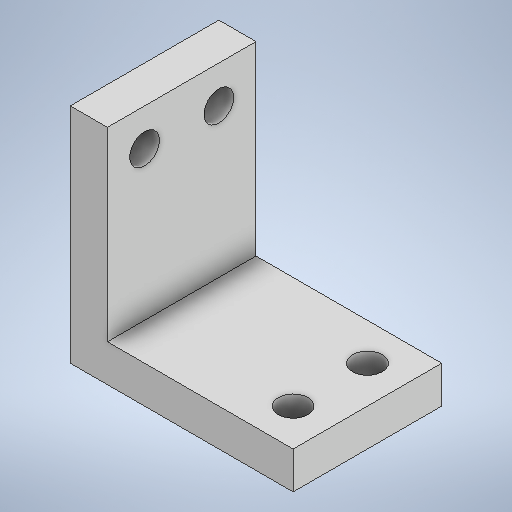
# Autodesk Inventor part: Fastener
Saved by Autodesk Inventor 2025.3 (Build 293356030, 356C)
## iProperties
Created: 2026-06-29
Part Number: Fastener
Material: Generic
Document SubType Name: Modeling
Designer: user
Density: 1 g/cm^3
Appearance: Default
Author: user
Autodesk Inventor part; units mm, degrees
ref_plane "YZ Plane" through (0, 0, 0) normal (1, 0, 0) x (0, 1, 0)
ref_plane "XZ Plane" through (0, 0, 0) normal (0, 1, 0) x (-1, 0, 0)
ref_plane "XY Plane" through (0, 0, 0) normal (0, 0, 1) x (1, 0, 0)
sketch "Sketch1" plane through (0, 0, 0) normal (0, 1, 0) x (-1, 0, 0)
  line L0 (0, 0) -> (-30, 0)
  line L1 (-30, 0) -> (-30, -20)
  line L2 (-30, -20) -> (0, -20)
  line L3 (0, -20) -> (0, 0)
  line L4 (0, 0) -> (-5, 0)
  line L5 (-15, -20) -> (0, -20)
  line L6 (0, -20) -> (0, 0)
  line L7 (-5, 0) -> (-5, -20)
  point P0 (-5, -20)
  dimension "d1" = 20
  dimension "d7" = 5
  dimension "d8" = 25
  constraints: 16 end point, 3 parallel, 2 horizontal, 2 perpendicular, 2 point on line, 1 midpoint
  measures "d1" distance of L1.end L0.end
  measures "d7" distance between parallel lines of L7 L3
  measures "d8" distance between parallel lines of L1 L7
extrude "Extrusion1" add sketch "Sketch1" along normal blind 30 contours L3 L2 L7 L0
extrude "Extrusion3" add sketch "Sketch1" along normal blind 5 contours L7 L2 L1 L0
sketch "Sketch2" plane through (0, 5, 0) normal (0, 1, 0) x (1, 0, 0)
  line L0 (5, 0) -> (5, 20) projected
  line L1 (5, 0) -> (30, 0) projected
  point P0 (0, 0)
  point P1 (25, 5)
  point P2 (25, 15)
  dimension "d18" = 20
  dimension "d19" = 10
  dimension "d20" = 20
  dimension "d21" = 5
  measures "d18" distance from line of L0 point (25, 5)
  measures "d19" distance of point (25, 15) point (25, 5)
  measures "d20" distance from line of L0 point (25, 15)
  measures "d21" distance from line of L1 point (25, 5)
hole "Hole1" at (25, 5, -5) at (25, 5, -15) direction (0, -1, 0) diameter 4 end through all
sketch "Sketch3" plane through (5, 30, 0) normal (1, 0, 0) x (0, 0, -1)
  line L0 (20, -25) -> (20, 0) projected
  line L1 (0, 0) -> (20, 0) projected
  line L2 (0, -25) -> (20, -25) projected
  point P0 (0, -30)
  point P1 (5, -5)
  point P2 (15, -5)
  point P3 (20, -12.5)
  dimension "d29" = 10
  dimension "d30" = 5
  dimension "d31" = 5
  dimension "d32" = 20
  constraints: 1 midpoint
  measures "d29" distance of point (15, -5) point (5, -5)
  measures "d30" horizontal distance of point (20, -12.5) point (15, -5)
  measures "d31" distance from line of L1 point (5, -5)
  measures "d32" distance from line of L2 point (15, -5)
hole "Hole2" at (5, 25, -5) at (5, 25, -15) direction (-1, 0, 0) diameter 4 end through all
body "Solid1"
